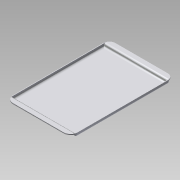
# Autodesk Inventor part: food tray
Saved by Autodesk Inventor 2015 (Build 190159000, 159)
## iProperties
Created: 2015-05-22
Part Number: food tray
Material: Aluminum 6061
Document SubType Name: Modeling
Designer: Joe Sheldon
Density: 2.7 g/cm^3
Appearance: Aluminum - Flat
Author: Joe Sheldon
Autodesk Inventor part; units mm, degrees
ref_plane "YZ Plane" through (0, 0, 0) normal (1, 0, 0) x (0, 1, 0)
ref_plane "XZ Plane" through (0, 0, 0) normal (0, 1, 0) x (-1, 0, 0)
ref_plane "XY Plane" through (0, 0, 0) normal (0, 0, 1) x (1, 0, 0)
sketch "Sketch1" plane through (0, 0, 0) normal (0, 1, 0) x (-1, 0, 0)
  line L0 (-114.3, 165.1) -> (114.3, 165.1)
  line L1 (114.3, 165.1) -> (114.3, -165.1)
  line L2 (114.3, -165.1) -> (-114.3, -165.1)
  line L3 (-114.3, -165.1) -> (-114.3, 165.1)
  line L4 (-114.3, 165.1) -> (114.3, -165.1) construction
  line L5 (114.3, 165.1) -> (-114.3, -165.1) construction
  point P0 (0, 0)
  dimension "d0" = 228.6
  dimension "d1" = 330.2
  constraints: 12 end point, 2 midpoint, 2 parallel, 1 horizontal, 1 perpendicular
  measures "d0" distance of L1.end L2.end
  measures "d1" distance of L0.end L1.end
extrude "Extrusion1" add sketch "Sketch1" along normal blind 1.5875
sketch "Sketch2" plane through (0, 0, 0) normal (0, -1, 0) x (1, 0, 0)
  line L0 (114.3, 165.1) -> (-114.3, 165.1) projected
  line L1 (-114.3, 165.1) -> (-114.3, -165.1) projected
  line L2 (-114.3, -165.1) -> (114.3, -165.1) projected
  line L3 (114.3, -165.1) -> (114.3, 165.1) projected
  line L4 (116.4167, 167.2167) -> (-116.4167, 167.2167)
  line L5 (-116.4167, 167.2167) -> (-116.4167, -167.2167)
  line L6 (-116.4167, -167.2167) -> (116.4167, -167.2167)
  line L7 (116.4167, -167.2167) -> (116.4167, 167.2167)
  point P0 (0, 0)
  dimension "d4" = 2.1167
  constraints: 8 end point, 3 other
  measures "d4" distance between parallel lines of L3 L7
extrude "Extrusion2" add sketch "Sketch2" against normal blind 12.7
sketch "Sketch3" plane through (-116.4167, 0, 167.2167) normal (0, 0, 1) x (1, 0, 0)
  line L0 (232.8333, 0) -> (0, 0) projected
  line L1 (232.8333, 0) -> (232.8333, 12.7) projected
  line L2 (0, 12.7) -> (232.8333, 12.7) projected
  line L3 (0, 0) -> (0, 12.7) projected
  line L4 (0, 0) -> (0, 12.7) projected
  line L5 (232.8333, 12.7) -> (0, 12.7)
  line L6 (0, 12.7) -> (0, 9.525)
  line L7 (0, 9.525) -> (232.8333, 9.525)
  line L8 (232.8333, 9.525) -> (232.8333, 12.7)
  point P0 (116.4167, 0)
  dimension "d7" = 3.175
  constraints: 8 end point, 2 parallel, 1 horizontal, 1 perpendicular, 1 point on line
  measures "d7" distance of L6.end L5.end
extrude "Extrusion3" add sketch "Sketch3" along normal blind 19.05 contours L7 L3 L2 L1
fillet "Fillet1" radius 25.4 2 edges at (116.4167, 11.1125, 186.2667) (-116.4167, 11.1125, 186.2667)
fillet "Fillet2" radius 6.35 6 edges at (116.2142, 0, 164.0672) (116.4167, 0, -3.175) (0, 0, 167.2167) (-116.2142, 0, 164.0672) (-116.4167, 0, -3.175) (0, 0, -167.2167)
fillet "Fillet3" radius 6.35 4 edges at (-114.3, 1.5875, 0) (0, 1.5875, 165.1) (0, 1.5875, -165.1) (114.3, 1.5875, 0)
fillet "Fillet4" radius 6.35 1 edges at (0, 12.7, 165.1)
mirror "Mirror1" about plane through (0, 0, 0) normal (0, 0, 1) of "Extrusion3"
fillet "Fillet5" radius 6.35 1 edges at (0, 12.7, -165.1)
fillet "Fillet6" radius 22.225 2 edges at (-116.4167, 11.1125, -186.2667) (116.4167, 11.1125, -186.2667)
body "Solid1"
